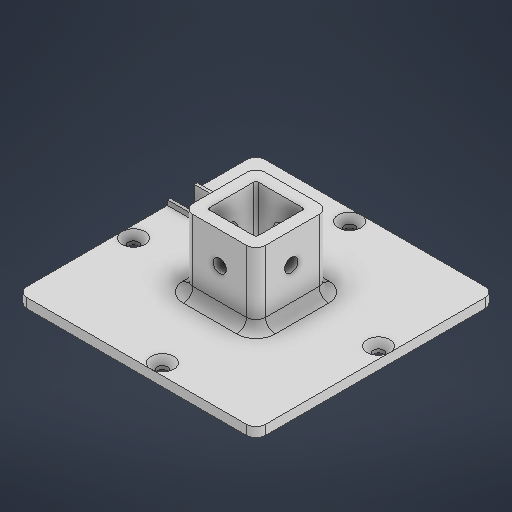
# Autodesk Inventor part: Lid
Saved by Autodesk Inventor 2025 (Build 290162010, 162A)
## iProperties
Created: 2024-10-14
Part Number: Lid
Material: Generic
Document SubType Name: Modeling
Designer: tzu98
Density: 1 g/cm^3
Appearance: Default
Author: tzu98
Autodesk Inventor part; units mm, degrees
ref_plane "YZ Plane" through (0, 0, 0) normal (1, 0, 0) x (0, 1, 0)
ref_plane "XZ Plane" through (0, 0, 0) normal (0, 1, 0) x (-1, 0, 0)
ref_plane "XY Plane" through (0, 0, 0) normal (0, 0, 1) x (1, 0, 0)
sketch "Sketch1" plane through (0, 0, 0) normal (0, 0, 1) x (1, 0, 0)
  line L0 (-49.7, 49.7) -> (49.7, 49.7)
  line L1 (49.7, 49.7) -> (49.7, -49.7)
  line L2 (49.7, -49.7) -> (-49.7, -49.7)
  line L3 (-49.7, -49.7) -> (-49.7, 49.7)
  line L4 (-49.7, 49.7) -> (49.7, -49.7) construction
  line L5 (49.7, 49.7) -> (-49.7, -49.7) construction
  line L6 (44, -44) -> (-44, -44)
  line L7 (-44, -44) -> (-44, 44)
  line L8 (-44, 44) -> (44, 44)
  line L9 (44, 44) -> (44, -44)
  line L10 (44, -44) -> (-44, 44) construction
  line L11 (-44, -44) -> (44, 44) construction
  circle A0 centre (-44, 44) radius 1.75
  circle A1 centre (44, 44) radius 1.75
  circle A2 centre (-44, -44) radius 1.75
  circle A3 centre (44, -44) radius 1.75
  point P0 (0, 0)
  dimension "d0" = 99.4
  dimension "d1" = 99.4
  dimension "d2" = 88
  dimension "d3" = 88
  dimension "d4" = 3.5
  dimension "d5" = 3.5
  dimension "d6" = 3.5
  dimension "d7" = 3.5
  constraints: 24 end point, 4 centre point, 4 coincident, 4 midpoint, 4 parallel, 2 horizontal, 2 perpendicular
  measures "d0" distance of L1.end L2.end
  measures "d1" distance of L0.end L1.end
  measures "d2" distance of L7.end L8.end
  measures "d3" distance of L6.end L7.end
  measures "d4" diameter of A0
  measures "d5" diameter of A1
  measures "d6" diameter of A2
  measures "d7" diameter of A3
extrude "Extrusion1" add sketch "Sketch1" along normal blind 4 contours L0 L1 L2 L3 | A2 L7 L6 | A2 L7 A0 L8 A1 L9 A3 L6 | L6 L7 A2 | A3 L9 L6 | L6 L9 A3 | A0 L8 L7 | L7 L8 A0 | A1 L8 L9 | L9 L8 A1
fillet "Fillet1" radius 4 4 edges at (-49.7, -49.7, 2) (49.7, -49.7, 2) (-49.7, 49.7, 2) (49.7, 49.7, 2)
sketch "Sketch2" plane through (0, 0, 4) normal (0, 0, 1) x (1, 0, 0)
  line L0 (10.125, -10.125) -> (-10.125, -10.125)
  line L1 (-10.125, -10.125) -> (-10.125, 10.125)
  line L2 (-10.125, 10.125) -> (10.125, 10.125)
  line L3 (10.125, 10.125) -> (10.125, -10.125)
  line L4 (10.125, -10.125) -> (-10.125, 10.125) construction
  line L5 (-10.125, -10.125) -> (10.125, 10.125) construction
  line L6 (-15.125, 15.125) -> (15.125, 15.125)
  line L7 (15.125, 15.125) -> (15.125, -15.125)
  line L8 (15.125, -15.125) -> (-15.125, -15.125)
  line L9 (-15.125, -15.125) -> (-15.125, 15.125)
  line L10 (-15.125, 15.125) -> (15.125, -15.125) construction
  line L11 (15.125, 15.125) -> (-15.125, -15.125) construction
  point P0 (0, 0)
  point P1 (0, -15.125)
  dimension "d15" = 20.25
  dimension "d16" = 20.25
  dimension "d17" = 5
  constraints: 24 end point, 5 midpoint, 4 parallel, 2 horizontal, 2 perpendicular, 1 point on line
  measures "d15" distance of L1.end L2.end
  measures "d16" distance of L0.end L1.end
  measures "d17" distance from line of point (0, -15.125) L0
extrude "Extrusion2" add sketch "Sketch2" along normal blind 30
fillet "Fillet3" radius 1 4 edges at (-10.125, -10.125, 19) (10.125, -10.125, 19) (10.125, 10.125, 19) (-10.125, 10.125, 19)
fillet "Fillet4" radius 4 8 edges at (15.125, -15.125, 19) (15.125, 15.125, 19) (-15.125, 15.125, 19) (-15.125, -15.125, 19) (0, -15.125, 4) (15.125, 0, 4) (0, 15.125, 4) (-15.125, 0, 4)
sketch "Sketch3" plane through (15.125, -11.125, 34) normal (1, 0, 0) x (0, 0, -1)
  line L0 (30, 22.25) -> (26, 22.25) projected
  line L1 (0, 0) -> (26, 22.25)
  circle A0 centre (12.4937, 10.6917) radius 2.75
  point P0 (34, 11.125)
  dimension "d22" = 5.5
  constraints: 2 end point, 1 centre point, 1 coincident, 1 point on line
  measures "d22" diameter of A0
extrude "Extrusion3" cut sketch "Sketch3" against normal through all
sketch "Sketch4" plane through (-11.125, -15.125, 8) normal (0, -1, 0) x (1, 0, 0)
  line L0 (-4, 26) -> (0, 26) projected
  line L1 (0, 0) -> (22.25, 0) projected
  line L2 (0, 26) -> (22.25, 0)
  circle A0 centre (11.125, 13) radius 2.75
  point P0 (11.125, -8)
  point P1 (9.337, 15.0894)
  point P2 (12.913, 10.9106)
  dimension "d25" = 5.5
  constraints: 2 end point, 1 centre point, 1 midpoint
  measures "d25" diameter of A0
extrude "Extrusion4" cut sketch "Sketch4" against normal through all
sketch "Sketch5" plane through (0, 0, 4) normal (0, 0, 1) x (1, 0, 0)
  line L0 (-43.5, 24) -> (-33.5, 24)
  line L1 (-33.5, 24) -> (-33.5, 14)
  line L2 (-33.5, 14) -> (-43.5, 14)
  line L3 (-43.5, 14) -> (-43.5, 24)
  line L4 (-48.7, 44.7) -> (-48.7, -44.7) projected
  line L5 (44.7, 48.7) -> (-44.7, 48.7) projected
  line L6 (-49.7, 45.7) -> (-49.7, -45.7) projected
  point P0 (0, 0)
  point P1 (-49.3, 43.8338)
  point P2 (-49.3, -43.8338)
  point P3 (43.8338, 49.3)
  point P4 (-43.8338, 49.3)
  dimension "d31" = 10
  dimension "d32" = 10
  dimension "d33" = 24.7
  dimension "d57" = 6.2
  constraints: 8 end point, 2 parallel, 1 horizontal, 1 perpendicular, 2 other
  measures "d31" distance between parallel lines of L0 L2
  measures "d32" distance between parallel lines of L3 L1
  measures "d57" distance between parallel lines of L6 L3
extrude "Extrusion5" cut sketch "Sketch5" against normal blind 10
fillet "Fillet5" radius 2 4 edges at (-43.5, 24, 2) (-33.5, 24, 2) (-33.5, 14, 2) (-43.5, 14, 2)
sketch "Sketch6" plane through (0, 0, 4) normal (0, 0, 1) x (1, 0, 0)
  line L0 (-41.5, 14) -> (-35.5, 14) projected
  line L1 (-41.5, 14) -> (-49.7, 14)
  line L2 (-49.7, 14) -> (-49.7, 24)
  line L3 (-49.7, 24) -> (-41.5, 24)
  line L4 (-41.5, 24) -> (-41.5, 14)
  line L5 (-49.7, 45.7) -> (-49.7, -45.7) projected
  point P0 (0, 0)
  point P1 (-35.5, 24)
  point P2 (-49.3, 43.8338)
  point P3 (-49.3, -43.8338)
  constraints: 8 end point, 2 parallel, 2 point on line, 1 horizontal, 1 perpendicular
extrude "Extrusion6" cut sketch "Sketch6" against normal blind 10
sketch "Sketch7" plane through (0, 0, 4) normal (0, 0, 1) x (1, 0, 0)
  arc A0 (11.125, -19.125) -> (19.125, -11.125) centre (11.125, -11.125) ccw projected
  line L0 (-11.125, -19.125) -> (11.125, -19.125) projected
  arc A1 (-19.125, -11.125) -> (-11.125, -19.125) centre (-11.125, -11.125) ccw projected
  line L1 (-19.125, 11.125) -> (-19.125, -11.125) projected
  arc A2 (-11.125, 19.125) -> (-19.125, 11.125) centre (-11.125, 11.125) ccw projected
  line L2 (11.125, 19.125) -> (-11.125, 19.125) projected
  arc A3 (19.125, 11.125) -> (11.125, 19.125) centre (11.125, 11.125) ccw projected
  line L3 (19.125, -11.125) -> (19.125, 11.125) projected
  line L4 (-35.5, 14) -> (-49.7, 14) projected
  line L5 (-49.7, 14) -> (-49.7, -45.7) projected
  arc A4 (-49.7, -45.7) -> (-45.7, -49.7) centre (-45.7, -45.7) ccw projected
  line L6 (-45.7, -49.7) -> (45.7, -49.7) projected
  arc A5 (45.7, -49.7) -> (49.7, -45.7) centre (45.7, -45.7) ccw projected
  line L7 (49.7, -45.7) -> (49.7, 45.7) projected
  arc A6 (49.7, 45.7) -> (45.7, 49.7) centre (45.7, 45.7) ccw projected
  line L8 (45.7, 49.7) -> (-45.7, 49.7) projected
  arc A7 (-45.7, 49.7) -> (-49.7, 45.7) centre (-45.7, 45.7) ccw projected
  line L9 (-49.7, 24) -> (-35.5, 24) projected
  arc A8 (-33.5, 22) -> (-35.5, 24) centre (-35.5, 22) ccw projected
  line L10 (-33.5, 22) -> (-33.5, 16) projected
  arc A9 (-35.5, 14) -> (-33.5, 16) centre (-35.5, 16) ccw projected
  line L11 (-49.7, 12.8) -> (-32.3, 12.8)
  line L12 (-32.3, 12.8) -> (-32.3, 25.2)
  line L13 (-32.3, 25.2) -> (-49.7, 25.2)
  line L14 (-49.7, 25.2) -> (-49.7, 12.8)
  line L15 (-49.7, 45.7) -> (-49.7, 24) projected
  point P0 (0, 0)
  point P1 (-42.6, 24)
  dimension "d40" = 1.2
  dimension "d41" = 1.2
  dimension "d42" = 1.2
  constraints: 8 end point, 2 parallel, 1 horizontal, 1 midpoint, 1 perpendicular, 1 point on line
  measures "d40" distance between parallel lines of L11 L4
  measures "d41" distance between parallel lines of L10 L12
  measures "d42" distance from line of point (-42.6, 24) L13
extrude "Extrusion7" add sketch "Sketch7" along normal blind 2 contours A9 L10 A8 L9 L14 L13 L12 L11 L5 L4
fillet "Fillet8" radius 2 2 edges at (-32.3, 25.2, 5) (-32.3, 12.8, 5)
sketch "Sketch8" plane through (0, 0, 4) normal (0, 0, 1) x (1, 0, 0)
  line L0 (45, 6.0205) -> (-45, 6.0205)
  line L1 (-45, 6.0205) -> (-45, -6.0205)
  line L2 (-45, -6.0205) -> (45, -6.0205)
  line L3 (45, -6.0205) -> (45, 6.0205)
  line L4 (45, 6.0205) -> (-45, -6.0205) construction
  line L5 (-45, 6.0205) -> (45, -6.0205) construction
  line L6 (6.0205, -45) -> (-6.0205, -45)
  line L7 (-6.0205, -45) -> (-6.0205, 45)
  line L8 (-6.0205, 45) -> (6.0205, 45)
  line L9 (6.0205, 45) -> (6.0205, -45)
  line L10 (6.0205, -45) -> (-6.0205, 45) construction
  line L11 (-6.0205, -45) -> (6.0205, 45) construction
  point P0 (0, 0)
  dimension "d46" = 90
  dimension "d47" = 12.041
  dimension "d48" = 12.041
  dimension "d49" = 90
  constraints: 24 end point, 4 midpoint, 4 parallel, 2 horizontal, 2 perpendicular
  measures "d46" distance of L1.end L2.end
  measures "d47" distance of L2.end L0.start
  measures "d48" distance of L7.end L8.end
  measures "d49" distance of L6.end L7.end
hole "Hole1" at (-45, -6.0205, 4) at (45, 6.0205, 4) at (6.0205, -45, 4) at (-6.0205, 45, 4) direction (0, 0, -1) diameter 4.3 end through all countersink diameter 9.4 countersink angle 90 clearance for "Countersunk Flat Head Screw DIN EN ISO 2009" size "M4" standard "DIN"
body "Solid1"
